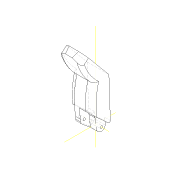
# Autodesk Inventor part: empty
Saved by Autodesk Inventor 2014 (Build 180170000, 170)
## iProperties
Created: 2015-04-13
Part Number: empty
Material: Generic
Document SubType Name: Modeling
Designer: Martin
Density: 1 g/cm^3
Appearance: Default
Author: Martin
Autodesk Inventor part; units mm, degrees
ref_plane "plane_support_bottom" through (-9, 0, 0) normal (-1, 0, 0) x (0, 0, 1)
ref_plane "plane_support_top" through (-4.75, -11.1852, 5.3387) normal (-1, 0, 0) x (0, 0.6427876, 0.7660444)
ref_plane "YZ Plane" through (0, 0, 0) normal (1, 0, 0) x (0, 1, 0)
sketch "Sketch1" plane through (0, 0, 0) normal (1, 0, 0) x (0, 1, 0)
  line L0 (-40.0242, 0) -> (72.7174, 0) projected
  line L1 (0, -18.7998) -> (0, 84.8204) projected
  circle A0 centre (0, 0) radius 1
  line L2 (0, 0) -> (-9.1925, 7.7135)
  circle A1 centre (-9.1925, 7.7135) radius 1
  line L3 (-4.5963, 3.8567) -> (-4.5963, 39.0567) construction
  line L4 (-4.5963, 39.0567) -> (-20.3696, 61.5834) construction
  circle A2 centre (-9.1925, 7.7135) radius 3.1 construction
  circle A3 centre (0, 0) radius 3.1 construction
  line L5 (-11.1852, 5.3387) -> (-1.9926, -2.3747)
  line L6 (-11.2639, 39.0567) -> (1.7361, 39.0567) construction
  line L7 (3.1, 0) -> (1.7361, 39.0567)
  line L8 (2.7783, 9.2135) -> (-12.2217, 9.2135) construction
  arc A4 (-11.2639, 39.0567) -> (-12.2217, 9.2135) centre (56.6114, 21.9412) ccw
  line L9 (-18.2398, 63.0747) -> (-22.4994, 60.0921)
  arc A5 (-22.4994, 60.0921) -> (-11.2639, 39.0567) centre (21.3923, 70.0175) ccw
  line L10 (-18.2398, 63.0747) -> (1.7361, 39.0567)
  arc A6 (-12.2827, 7.4669) -> (-11.1852, 5.3387) centre (-9.1925, 7.7135) ccw
  arc A7 (-1.9926, -2.3747) -> (3.1, 0) centre (0, 0) ccw
  line L11 (-12.2827, 7.4669) -> (-12.2217, 9.2135)
  dimension "d0" = 2
  dimension "d1" = 12
  dimension "d2" = 40
  dimension "d4" = 27.5
  dimension "d5" = 145
  dimension "d7" = 6.2
  dimension "d9" = 92
  dimension "d12" = 13
  dimension "d13" = 35.2
  dimension "d14" = 15
  dimension "d15" = 70
  dimension "d16" = 5.2
  dimension "d17" = 45
  dimension "d21" = 1.5
  constraints: 20 end point, 12 point on circle, 8 centre point, 4 coincident, 4 equal radius, 3 parallel, 3 point on line, 2 midpoint, 2 perpendicular, 2 tangent
  measures "d0" diameter of A0
  measures "d1" distance of L2.start L2.end
  measures "d2" angle of L0 L2
  measures "d4" distance of L4.end L3.end
  measures "d5" angle of L3 L4
  measures "d7" diameter of A3
  measures "d9" angle of L0 L7
  measures "d12" distance of L6.start L6.end
  measures "d13" distance of L3.start L3.end
  measures "d14" distance of L8.start L8.end
  measures "d15" radius of A4
  measures "d16" distance of L9.start L9.end
  measures "d17" radius of A5
  measures "d21" distance from line of L8 A2.centre
extrude "ext_main_profile" add sketch "Sketch1" along normal mid plane 18 contours A0 L1 L10 L7 L0 | L0 A7 L1 A0 | A0 L1 A7 L5 L0 | L0 L5 A6 L11 A4 A5 L9 L10 L1 A0
sketch "Sketch2" plane through (0, 0, 0) normal (0, 1, 0) x (-1, 0, 0)
  line L0 (9, 63.0747) -> (-9, 63.0747) projected
  line L1 (-9, 39.0567) -> (-9, 63.0747) projected
  line L2 (9, 39.0567) -> (-9, 39.0567) projected
  line L3 (9, 63.0747) -> (9, 39.0567) projected
  line L4 (9, 39.0567) -> (-9, 39.0567) projected
  line L5 (0, -12.6149) -> (0, 75.6896) projected
  line L6 (-6.8987, 63.0747) -> (-9, 39.0567)
  line L7 (9, 39.0567) -> (6.8987, 63.0747)
  point P0 (0, 0)
  dimension "d22" = 5
  constraints: 4 end point, 2 point on line, 1 other
  measures "d22" angle of L1 L6
extrude "ext_cut_distal_lateralchanfer" [suppressed]
sketch "Sketch4" plane through (9, 0, 0) normal (1, 0, 0) x (0, 0, -1)
  line L0 (-5.3387, -11.1852) -> (2.3747, -1.9926) projected
  arc A0 (2.3747, -1.9926) -> (0, 3.1) centre (0, 0) ccw projected
  circle A1 centre (0, 0) radius 3.1 construction
  line L1 (-16.575, -13.3749) -> (-0.5054, 5.7762)
  line L2 (-0.5054, 5.7762) -> (5.7762, 0.5054)
  line L3 (5.7762, 0.5054) -> (-10.2935, -18.6458)
  line L4 (-10.2935, -18.6458) -> (-16.575, -13.3749)
  circle A2 centre (0, 0) radius 1 projected
  circle A3 centre (0, 0) radius 4.1 construction
  arc A4 (-39.0567, -11.2639) -> (-9.2135, -12.2217) centre (-21.9412, 56.6114) ccw projected
  line L5 (-0.5054, 5.7762) -> (-17.963, -13.2754)
  line L6 (-17.963, -13.2754) -> (-17.1312, -14.0377)
  line L7 (-17.1312, -14.0377) -> (-16.575, -13.3749)
  point P0 (-1.6668, -5.9095)
  point P1 (-9.9853, -12.3487)
  dimension "d31" = 1
  dimension "d38" = 25
  dimension "d51" = 2.5
  constraints: 14 end point, 4 perpendicular, 3 tangent, 2 centre point, 2 coincident, 1 collinear, 1 concentric, 1 point on circle, 2 other
  measures "d31" radial gap between concentric circles of A3 A1
  measures "d38" distance of L2.end L3.end
  measures "d51" angle of L1 L5
extrude "ext_cut_lateralfit" cut sketch "Sketch4" against normal blind 4.5 contours L7 L6 A4 L1 | L1 L2 L3 L4 | A4 L5 L1 | A2
fillet "fillet_lateralrelief" radius 1 1 edges at (6.75, 2.9933, 3.0554)
mirror "Mirror1" about plane through (0, 0, 0) normal (1, 0, 0) of "ext_cut_lateralfit", "fillet_lateralrelief"
sketch "Sketch5" plane through (4.5, 0, 0) normal (1, 0, 0) x (0, 0, -1)
  line L0 (2.3747, -1.9926) -> (-5.3387, -11.1852) projected
  circle A0 centre (0, 0) radius 1 projected
  circle A1 centre (-7.7135, -9.1925) radius 1 projected
  circle A2 centre (-7.7135, -9.1925) radius 4.1 construction
  line L1 (-8.2057, -5.1222) -> (0.647, -4.0516)
  circle A3 centre (0, 0) radius 4.1 construction
  line L2 (-10.8542, -6.5571) -> (-19.2105, -16.5157)
  line L3 (-19.2105, -16.5157) -> (-12.9289, -21.7865)
  line L4 (-12.9289, -21.7865) -> (3.1408, -2.6354)
  arc A4 (-8.2057, -5.1222) -> (-10.8542, -6.5571) centre (-7.7135, -9.1925) ccw
  arc A5 (0.647, -4.0516) -> (3.1408, -2.6354) centre (-0.0093, 0.0078) ccw
  line L5 (-17.963, -13.2754) -> (-4.6665, 1.2351) projected
  arc A6 (-9.271, -5.251) -> (-11.8016, -6.5514) centre (-8.7787, -9.3214) ccw
  line L6 (-17.963, -13.2754) -> (-4.6665, 1.2351) projected
  line L7 (-9.271, -5.251) -> (-8.2057, -5.1222)
  line L8 (-11.8016, -6.5514) -> (-20.1838, -15.699)
  line L9 (-20.1838, -15.699) -> (-19.2105, -16.5157)
  point P0 (-13.9612, -8.3044)
  point P1 (-12.5955, -11.0144)
  dimension "d52" = 8.2
  dimension "d35" = 25
  constraints: 14 end point, 8 point on circle, 5 tangent, 4 centre point, 4 point on line, 2 coincident, 2 perpendicular, 1 collinear, 1 concentric, 1 equal radius, 1 parallel, 7 other
  measures "d35" distance of L3.end L4.end
extrude "ext_linkfit" cut sketch "Sketch5" against normal blind 5 contours L1 A5 L4 L3 L2 A4 | A4 L2 L9 L8 L5 A6 L7
fillet "fillet_medial" radius 4.5 2 edges at (9, -13.0724, 28.5864) (-9, -13.0724, 28.5864)
fillet "fillet_distal" radius 2.7 4 edges at (9, -9.4191, 37.2203) (9, -18.3005, 48.8166) (-9, -9.4191, 37.2203) (-9, -18.3005, 48.8166)
sketch "Sketch6" plane through (-9, -18.2398, 63.0747) normal (0, 0.7688357, 0.6394464) x (1, 0, 0)
  line L0 (18, 31.2394) -> (18, 0) projected
  line L1 (0, 31.2394) -> (18, 31.2394) projected
  line L2 (0, 0) -> (0, 31.2394) projected
  line L3 (0, 4.8394) -> (18, 4.8394) construction
  line L4 (0, -0.8017) -> (18, -0.8017)
  line L5 (18, -0.8017) -> (18, 4.8394)
  line L6 (0, 4.8394) -> (0, -0.8017)
  arc A0 (0, 4.8394) -> (18, 4.8394) centre (9, 9.1983) ccw
  point P0 (9, 60.1575)
  point P1 (9, -0.8017)
  dimension "d42" = 26.4
  dimension "d43" = 10
  constraints: 8 end point, 3 point on circle, 2 perpendicular, 2 point on line, 1 centre point, 1 collinear, 1 midpoint, 1 parallel
  measures "d42" distance between parallel lines of L1 L3
  measures "d43" radius of A0
extrude "ext_cut_tip" cut sketch "Sketch6" against normal through all contours L0 L5 L4 A0 | L4 L6 L2 A0
sketch "Sketch7" plane through (-9, 0, 0) normal (-1, 0, 0) x (0, 0, 1)
  line L0 (5.0787, 2.9226) -> (0, 3.1) projected
  arc A0 (0, 3.1) -> (-2.3747, -1.9926) centre (0, 0) ccw projected
  line L1 (5.3387, -11.1852) -> (-2.3747, -1.9926) projected
  arc A1 (9.2135, -12.2217) -> (16.2036, -12.9323) centre (19.7786, 56.9764) ccw projected
  line L2 (1.4892, 3.048) -> (14.8668, -12.8948)
  line L3 (14.8668, -12.8948) -> (6.5289, -12.6036)
  line L4 (6.5289, -12.6036) -> (-4.3674, 0.3821)
  line L5 (-4.3674, 0.3821) -> (-1.0832, 3.1378)
  line L6 (-1.0832, 3.1378) -> (1.4892, 3.048)
  line L7 (16.2036, -12.9323) -> (4.2777, 1.2805) projected
  point P0 (0, 0)
  dimension "d48" = 1
  constraints: 10 end point, 3 collinear, 3 parallel, 2 tangent, 1 perpendicular
  measures "d48" distance between parallel lines of L2 L7
equation "\"d0\" = screw_m2_bore_selfthreading"
equation "\"d1\" = general_distal_linkbore_distance"
equation "\"d2\" = general_distal_linkbore_angle"
equation "\"d5\" = general_distal_medialdistal_angle"
equation "\"d7\" = general_bore_support_diameter"
equation "\"d12\" = general_distal_distalphalanx_thickness"
equation "\"d14\" = general_distal_medialphalanx_thickness"
equation "\"d16\" = 0.4 * general_distal_distalphalanx_thickness"
equation "\"d18\" = general_distal_width"
equation "\"d39\" = 0.25 * general_distal_width"
equation "\"d40\" = 0.15 * general_distal_width"
equation "\"d48\" = print_support_xy_clearance"
equation "\"d47\" = print_support_z_clearance"
equation "\"screw_m2_bore_selfthreading\" = 2"
equation "\"general_distal_linkbore_distance\" = 12"
equation "\"general_distal_linkbore_angle\" = 40deg"
equation "\"general_distal_medialdistal_angle\" = 145deg"
equation "\"general_bore_support_diameter\" = 6.2"
equation "\"general_distal_distalphalanx_thickness\" = 13"
equation "\"general_distal_medialphalanx_thickness\" = 15"
equation "\"general_distal_width\" = 18"
equation "\"print_support_xy_clearance\" = 1"
equation "\"print_support_z_clearance\" = 0.4"
body "Solid1"
